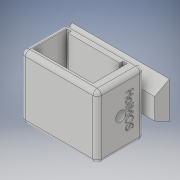
# Autodesk Inventor part: 7.2 Schienenläufer
Saved by Autodesk Inventor 2018.3 (Build 223284000, 284)
## iProperties
Created: 2018-10-11
Part Number: 7.2 Schienenläufer
Material: Generisch
Document SubType Name: Modeling
Designer: pgmadmin
Density: 1 g/cm^3
Appearance: Vorgabe
Author: pgmadmin
Autodesk Inventor part; units mm, degrees
ref_plane "YZ Plane" through (0, 0, 0) normal (1, 0, 0) x (0, 1, 0)
ref_plane "XZ Plane" through (0, 0, 0) normal (0, 1, 0) x (-1, 0, 0)
ref_plane "XY Plane" through (0, 0, 0) normal (0, 0, 1) x (1, 0, 0)
sketch "Skizze1" plane through (0, 0, 0) normal (0, 0, 1) x (1, 0, 0)
  line L0 (-14.1284, 0) -> (-14.1284, 16.2)
  line L1 (-14.1284, 16.2) -> (-12.1284, 16.2)
  line L2 (-12.1284, 16.2) -> (-12.1284, 1.6)
  line L3 (-12.1284, 1.6) -> (12.3716, 1.6)
  line L4 (12.3716, 1.6) -> (12.3716, 16.2)
  line L5 (12.3716, 16.2) -> (14.3716, 16.2)
  line L6 (14.3716, 16.2) -> (14.3716, 0)
  line L7 (14.3716, 0) -> (-14.1284, 0)
  line L8 (-16.6284, 19.2) -> (19.3716, 19.2)
  line L9 (19.3716, 19.2) -> (19.3716, -3)
  line L10 (19.3716, -3) -> (-16.6284, -3)
  line L11 (-16.6284, -3) -> (-16.6284, 19.2)
  line L12 (-12.1284, 14.7) -> (12.3716, 14.7)
  point P0 (0, 0)
  dimension "d1" = 2
  dimension "d3" = 2
  dimension "d4" = 1.6
  dimension "d5" = 3
  dimension "d7" = 2.5
  dimension "d8" = 5
  dimension "d9" = 1.5
  dimension "d26" = 3
  dimension "d27" = 28.5
  dimension "d28" = 16.2
  constraints: 26 end point, 8 perpendicular, 4 point on line, 2 parallel, 1 horizontal, 1 vertical
  measures "d1" distance of L0.end L1.end
  measures "d3" distance of L4.end L5.end
  measures "d4" distance between parallel lines of L3 L7
  measures "d5" distance between parallel lines of L10 L7
  measures "d7" distance between parallel lines of L11 L0
  measures "d8" distance between parallel lines of L9 L6
  measures "d9" distance of L1.end L12.start
  measures "d26" distance between parallel lines of L8 L1
  measures "d27" distance of L6.end L0.start
  measures "d28" distance of L0.start L0.end
extrude "Extrusion1" add sketch "Skizze1" along normal blind 30
fillet "Rundung1" radius 2 12 edges at (19.3716, 19.2, 15) (19.3716, -3, 15) (-16.6284, -3, 15) (-16.6284, 19.2, 15) (1.3716, 19.2, 30) (-16.6284, 8.1, 30) (1.3716, -3, 30) (19.3716, 8.1, 30) (19.3716, 8.1, 0) (1.3716, -3, 0) (1.3716, 19.2, 0) (-16.6284, 8.1, 0)
sketch "Skizze2" plane through (19.3716, -1, 28) normal (1, 0, 0) x (0, 0, -1)
  line L0 (0, 20.2) -> (26, 20.2) projected
  line L1 (8, 20.2) -> (4.25, 27.2)
  line L2 (4.25, 27.2) -> (21.75, 27.2)
  line L3 (21.75, 27.2) -> (18, 20.2)
  line L4 (28, 0) -> (28, 18.2) projected
  point P0 (28, 1)
  dimension "d13" = 10
  dimension "d15" = 7
  dimension "d16" = 3.75
  dimension "d17" = 3.75
  dimension "d18" = 17.5
  dimension "d19" = 10
  constraints: 6 end point, 2 point on line, 1 parallel
  measures "d13" distance of L3.end L1.start
  measures "d15" vertical distance of L1.end L1.start
  measures "d16" horizontal distance of L2.end L3.end
  measures "d17" horizontal distance of L1.start L1.end
  measures "d18" distance of L1.end L2.end
  measures "d19" distance from line of L4 L3.end
extrude "Extrusion2" add sketch "Skizze2" against normal blind 41 and the other way blind 5
sketch "Skizze5" plane through (19.3716, -1, 28) normal (1, 0, 0) x (0, 0, -1)
  circle A0 centre (13, 9.1) radius 2.4
  line L0 (13, 9.1) -> (-2, 9.1)
  line L1 (-2, 18.2) -> (-2, 0) projected
  line L2 (13, 9.1) -> (13, 20.2)
  line L3 (8, 20.2) -> (18, 20.2) projected
  line L4 (13, 9.1) -> (28, 9.1)
  point P0 (28, 1)
  dimension "d31" = 4.8
  dimension "d32" = 90
  dimension "d35" = 15
  constraints: 6 end point, 2 midpoint, 1 centre point, 1 collinear, 1 horizontal, 1 vertical
  measures "d31" diameter of A0
  measures "d32" angle of L2 L0
  measures "d35" distance between parallel lines of L1 L2
extrude "Extrusion5" cut sketch "Skizze5" against normal blind 10
sketch "Skizze6" plane through (19.3716, -1, 28) normal (1, 0, 0) x (0, 0, -1)
  circle A0 centre (13, 9.1) radius 2.4 projected
  line L0 (13, 11.5) -> (-2, 11.5)
  line L1 (-2, 18.2) -> (-2, 0) projected
  line L2 (28, 0) -> (28, 18.2) projected
  line L3 (28, 11.5) -> (13, 11.5)
  line L4 (0, -2) -> (26, -2) projected
  line L5 (6.9088, 11.5) -> (6.4437, 11.5)
  line L6 (6.4437, 11.5) -> (6.4437, 13.2131)
  line L7 (6.4437, 13.2131) -> (4.8327, 13.2131)
  line L8 (4.8327, 13.2131) -> (4.8327, 11.5)
  line L9 (4.8327, 11.5) -> (4.3675, 11.5)
  line L10 (4.3675, 11.5) -> (4.3675, 15)
  line L11 (4.3675, 15) -> (4.8327, 15)
  line L12 (4.8327, 15) -> (4.8327, 13.6272)
  line L13 (4.8327, 13.6272) -> (6.4437, 13.6272)
  line L14 (6.4437, 13.6272) -> (6.4437, 15)
  line L15 (6.4437, 15) -> (6.9088, 15)
  line L16 (6.9088, 15) -> (6.9088, 11.5)
  spline S0 degree 2 poles (9.7423, 12.8132) (9.7423, 12.1495) (9.1041, 11.4263) (8.5709, 11.4263) knots 0 0 0 1 2 2 2
  spline S1 degree 2 poles (8.5709, 11.4263) (8.0235, 11.4263) (7.3967, 12.1722) (7.3967, 12.8132) knots 0 0 0 1 2 2 2
  spline S2 degree 2 poles (7.3967, 12.8132) (7.3967, 13.4712) (8.0434, 14.2002) (8.5709, 14.2002) knots 0 0 0 1 2 2 2
  spline S3 degree 2 poles (8.5709, 14.2002) (9.1041, 14.2002) (9.7423, 13.4741) (9.7423, 12.8132) knots 0 0 0 1 2 2 2
  spline S4 degree 2 poles (9.2857, 12.8132) (9.2857, 13.3237) (8.9141, 13.8201) (8.5709, 13.8201) knots 0 0 0 1 2 2 2
  spline S5 degree 2 poles (8.5709, 13.8201) (8.2277, 13.8201) (7.8533, 13.3237) (7.8533, 12.8132) knots 0 0 0 1 2 2 2
  spline S6 degree 2 poles (7.8533, 12.8132) (7.8533, 12.3169) (8.2277, 11.8063) (8.5709, 11.8063) knots 0 0 0 1 2 2 2
  spline S7 degree 2 poles (8.5709, 11.8063) (8.9113, 11.8063) (9.2857, 12.3083) (9.2857, 12.8132) knots 0 0 0 1 2 2 2
  line L17 (10.6471, 11.5) -> (10.2046, 11.5)
  line L18 (10.2046, 11.5) -> (10.2046, 15.156)
  line L19 (10.2046, 15.156) -> (10.6471, 15.156)
  line L20 (10.6471, 15.156) -> (10.6471, 11.5)
  line L21 (14.3314, 11.5) -> (13.8663, 11.5)
  line L22 (13.8663, 11.5) -> (13.8663, 14.515)
  line L23 (13.8663, 14.515) -> (12.953, 12.4643)
  line L24 (12.953, 12.4643) -> (12.6694, 12.4643)
  line L25 (12.6694, 12.4643) -> (11.7646, 14.515)
  line L26 (11.7646, 14.515) -> (11.7646, 11.5)
  line L27 (11.7646, 11.5) -> (11.3306, 11.5)
  line L28 (11.3306, 11.5) -> (11.3306, 15)
  line L29 (11.3306, 15) -> (11.966, 15)
  line L30 (11.966, 15) -> (12.8395, 13.0515)
  line L31 (12.8395, 13.0515) -> (13.6848, 15)
  line L32 (13.6848, 15) -> (14.3314, 15)
  line L33 (14.3314, 15) -> (14.3314, 11.5)
  spline S8 degree 2 poles (17.5166, 14.6001) (17.7152, 14.3675) (17.9364, 13.6868) (17.9364, 13.25) knots 0 0 0 1 2 2 2
  spline S9 degree 2 poles (17.9364, 13.25) (17.9364, 12.8246) (17.7208, 12.1353) (17.5166, 11.9028) knots 0 0 0 1 2 2 2
  spline S10 degree 2 poles (17.5166, 11.9028) (17.3011, 11.6588) (16.731, 11.4263) (16.3878, 11.4263) knots 0 0 0 1 2 2 2
  spline S11 degree 2 poles (16.3878, 11.4263) (16.0332, 11.4263) (15.466, 11.6673) (15.2589, 11.9028) knots 0 0 0 1 2 2 2
  spline S12 degree 2 poles (15.2589, 11.9028) (15.0575, 12.1353) (14.842, 12.8189) (14.842, 13.25) knots 0 0 0 1 2 2 2
  spline S13 degree 2 poles (14.842, 13.25) (14.842, 13.6896) (15.0604, 14.359) (15.2618, 14.6001) knots 0 0 0 1 2 2 2
  spline S14 degree 2 poles (15.2618, 14.6001) (15.466, 14.8327) (16.0361, 15.0737) (16.3878, 15.0737) knots 0 0 0 1 2 2 2
  spline S15 degree 2 poles (16.3878, 15.0737) (16.7451, 15.0737) (17.3181, 14.8241) (17.5166, 14.6001) knots 0 0 0 1 2 2 2
  spline S16 degree 2 poles (17.4514, 13.25) (17.4514, 13.596) (17.3011, 14.1321) (17.1649, 14.3079) knots 0 0 0 1 2 2 2
  spline S17 degree 2 poles (17.1649, 14.3079) (17.0259, 14.4895) (16.6345, 14.671) (16.3906, 14.671) knots 0 0 0 1 2 2 2
  spline S18 degree 2 poles (16.3906, 14.671) (16.1382, 14.671) (15.7581, 14.4951) (15.6135, 14.3079) knots 0 0 0 1 2 2 2
  spline S19 degree 2 poles (15.6135, 14.3079) (15.4745, 14.1293) (15.327, 13.5904) (15.327, 13.25) knots 0 0 0 1 2 2 2
  spline S20 degree 2 poles (15.327, 13.25) (15.327, 12.5608) (15.9056, 11.829) (16.3906, 11.829) knots 0 0 0 1 2 2 2
  spline S21 degree 2 poles (16.3906, 11.829) (16.8756, 11.829) (17.4514, 12.5608) (17.4514, 13.25) knots 0 0 0 1 2 2 2
  spline S22 degree 2 poles (19.4226, 11.4376) (19.0425, 11.4376) (18.5093, 11.5964) (18.2739, 11.7099) knots 0 0 0 1 2 2 2
  line L34 (18.2739, 11.7099) -> (18.2739, 12.2942)
  line L35 (18.2739, 12.2942) -> (18.3079, 12.2942)
  spline S23 degree 2 poles (18.3079, 12.2942) (18.5377, 12.0786) (19.1191, 11.8404) (19.3886, 11.8404) knots 0 0 0 1 2 2 2
  spline S24 degree 2 poles (19.3886, 11.8404) (19.7743, 11.8404) (20.1686, 12.1609) (20.1686, 12.4246) knots 0 0 0 1 2 2 2
  spline S25 degree 2 poles (20.1686, 12.4246) (20.1686, 12.6345) (19.9615, 12.8955) (19.7374, 12.9607) knots 0 0 0 1 2 2 2
  spline S26 degree 2 poles (19.7374, 12.9607) (19.5758, 13.0061) (19.3063, 13.0685) (19.1049, 13.1195) knots 0 0 0 1 2 2 2
  spline S27 degree 2 poles (19.1049, 13.1195) (18.9234, 13.1677) (18.637, 13.3124) (18.5263, 13.4287) knots 0 0 0 1 2 2 2
  spline S28 degree 2 poles (18.5263, 13.4287) (18.4186, 13.545) (18.2994, 13.857) (18.2994, 14.0612) knots 0 0 0 1 2 2 2
  spline S29 degree 2 poles (18.2994, 14.0612) (18.2994, 14.4866) (18.9631, 15.0624) (19.4765, 15.0624) knots 0 0 0 1 2 2 2
  spline S30 degree 2 poles (19.4765, 15.0624) (19.7715, 15.0624) (20.2934, 14.9461) (20.5174, 14.8355) knots 0 0 0 1 2 2 2
  line L36 (20.5174, 14.8355) -> (20.5174, 14.2796)
  line L37 (20.5174, 14.2796) -> (20.4834, 14.2796)
  spline S31 degree 2 poles (20.4834, 14.2796) (20.316, 14.4327) (19.7942, 14.6596) (19.5077, 14.6596) knots 0 0 0 1 2 2 2
  spline S32 degree 2 poles (19.5077, 14.6596) (19.1844, 14.6596) (18.7844, 14.3562) (18.7844, 14.1094) knots 0 0 0 1 2 2 2
  spline S33 degree 2 poles (18.7844, 14.1094) (18.7844, 13.8882) (19.0199, 13.6244) (19.2411, 13.5648) knots 0 0 0 1 2 2 2
  spline S34 degree 2 poles (19.2411, 13.5648) (19.3886, 13.5251) (19.8169, 13.423) (19.9587, 13.3805) knots 0 0 0 1 2 2 2
  spline S35 degree 2 poles (19.9587, 13.3805) (20.3189, 13.2699) (20.6536, 12.8246) (20.6536, 12.4984) knots 0 0 0 1 2 2 2
  spline S36 degree 2 poles (20.6536, 12.4984) (20.6536, 12.2913) (20.4862, 11.8942) (20.3359, 11.7553) knots 0 0 0 1 2 2 2
  spline S37 degree 2 poles (20.3359, 11.7553) (20.1686, 11.6021) (19.7431, 11.4376) (19.4226, 11.4376) knots 0 0 0 1 2 2 2
  point P0 (28, 1)
  dimension "d36" = 13.5
  constraints: 4 end point, 3 point on line, 2 horizontal, 1 perpendicular, 1 vertical alignment, 1 other
  measures "d36" distance between parallel lines of L4 L0
extrude "Extrusion6" cut sketch "Skizze6" against normal blind 2 contours L0 L6 L7 L8 L10 L11 L12 L13 L14 L15 L16 | S0 S1 L0 | L0 S1 S2 S3 S0 | L0 L18 L19 L20 | S22 L34 L35 S23 S24 S25 S26 S27 S28 S29 S30 L36 L37 S31 S32 S33 S34 S35 S36 S37 L3 | L3 S37 S22 | S11 S12 S13 S14 S15 S8 S9 S10 L3 | L3 S10 S11 | L0 L28 L29 L30 L31 L32 L33 L3 L22 L23 L24 L25 L26
sketch "Skizze7" plane through (-16.6284, -1, 2) normal (-1, 0, 0) x (0, 0, 1)
  line L0 (0, 18.2) -> (0, 0) projected
  line L1 (0, 11.5) -> (25.983, 11.5)
  line L2 (0, -2) -> (26, -2) projected
  line L3 (8.9088, 11.5) -> (8.4437, 11.5)
  line L4 (8.4437, 11.5) -> (8.4437, 13.2131)
  line L5 (8.4437, 13.2131) -> (6.8327, 13.2131)
  line L6 (6.8327, 13.2131) -> (6.8327, 11.5)
  line L7 (6.8327, 11.5) -> (6.3675, 11.5)
  line L8 (6.3675, 11.5) -> (6.3675, 15)
  line L9 (6.3675, 15) -> (6.8327, 15)
  line L10 (6.8327, 15) -> (6.8327, 13.6272)
  line L11 (6.8327, 13.6272) -> (8.4437, 13.6272)
  line L12 (8.4437, 13.6272) -> (8.4437, 15)
  line L13 (8.4437, 15) -> (8.9088, 15)
  line L14 (8.9088, 15) -> (8.9088, 11.5)
  spline S0 degree 2 poles (11.7423, 12.8132) (11.7423, 12.1495) (11.1041, 11.4263) (10.5709, 11.4263) knots 0 0 0 1 2 2 2
  spline S1 degree 2 poles (10.5709, 11.4263) (10.0235, 11.4263) (9.3967, 12.1722) (9.3967, 12.8132) knots 0 0 0 1 2 2 2
  spline S2 degree 2 poles (9.3967, 12.8132) (9.3967, 13.4712) (10.0434, 14.2002) (10.5709, 14.2002) knots 0 0 0 1 2 2 2
  spline S3 degree 2 poles (10.5709, 14.2002) (11.1041, 14.2002) (11.7423, 13.4741) (11.7423, 12.8132) knots 0 0 0 1 2 2 2
  spline S4 degree 2 poles (11.2857, 12.8132) (11.2857, 13.3237) (10.9141, 13.8201) (10.5709, 13.8201) knots 0 0 0 1 2 2 2
  spline S5 degree 2 poles (10.5709, 13.8201) (10.2277, 13.8201) (9.8533, 13.3237) (9.8533, 12.8132) knots 0 0 0 1 2 2 2
  spline S6 degree 2 poles (9.8533, 12.8132) (9.8533, 12.3169) (10.2277, 11.8063) (10.5709, 11.8063) knots 0 0 0 1 2 2 2
  spline S7 degree 2 poles (10.5709, 11.8063) (10.9113, 11.8063) (11.2857, 12.3083) (11.2857, 12.8132) knots 0 0 0 1 2 2 2
  line L15 (12.6471, 11.5) -> (12.2046, 11.5)
  line L16 (12.2046, 11.5) -> (12.2046, 15.156)
  line L17 (12.2046, 15.156) -> (12.6471, 15.156)
  line L18 (12.6471, 15.156) -> (12.6471, 11.5)
  line L19 (16.3314, 11.5) -> (15.8663, 11.5)
  line L20 (15.8663, 11.5) -> (15.8663, 14.515)
  line L21 (15.8663, 14.515) -> (14.953, 12.4643)
  line L22 (14.953, 12.4643) -> (14.6694, 12.4643)
  line L23 (14.6694, 12.4643) -> (13.7646, 14.515)
  line L24 (13.7646, 14.515) -> (13.7646, 11.5)
  line L25 (13.7646, 11.5) -> (13.3306, 11.5)
  line L26 (13.3306, 11.5) -> (13.3306, 15)
  line L27 (13.3306, 15) -> (13.966, 15)
  line L28 (13.966, 15) -> (14.8395, 13.0515)
  line L29 (14.8395, 13.0515) -> (15.6848, 15)
  line L30 (15.6848, 15) -> (16.3314, 15)
  line L31 (16.3314, 15) -> (16.3314, 11.5)
  spline S8 degree 2 poles (19.5166, 14.6001) (19.7152, 14.3675) (19.9364, 13.6868) (19.9364, 13.25) knots 0 0 0 1 2 2 2
  spline S9 degree 2 poles (19.9364, 13.25) (19.9364, 12.8246) (19.7208, 12.1353) (19.5166, 11.9028) knots 0 0 0 1 2 2 2
  spline S10 degree 2 poles (19.5166, 11.9028) (19.3011, 11.6588) (18.731, 11.4263) (18.3878, 11.4263) knots 0 0 0 1 2 2 2
  spline S11 degree 2 poles (18.3878, 11.4263) (18.0332, 11.4263) (17.466, 11.6673) (17.2589, 11.9028) knots 0 0 0 1 2 2 2
  spline S12 degree 2 poles (17.2589, 11.9028) (17.0575, 12.1353) (16.842, 12.8189) (16.842, 13.25) knots 0 0 0 1 2 2 2
  spline S13 degree 2 poles (16.842, 13.25) (16.842, 13.6896) (17.0604, 14.359) (17.2618, 14.6001) knots 0 0 0 1 2 2 2
  spline S14 degree 2 poles (17.2618, 14.6001) (17.466, 14.8327) (18.0361, 15.0737) (18.3878, 15.0737) knots 0 0 0 1 2 2 2
  spline S15 degree 2 poles (18.3878, 15.0737) (18.7451, 15.0737) (19.3181, 14.8241) (19.5166, 14.6001) knots 0 0 0 1 2 2 2
  spline S16 degree 2 poles (19.4514, 13.25) (19.4514, 13.596) (19.3011, 14.1321) (19.1649, 14.3079) knots 0 0 0 1 2 2 2
  spline S17 degree 2 poles (19.1649, 14.3079) (19.0259, 14.4895) (18.6345, 14.671) (18.3906, 14.671) knots 0 0 0 1 2 2 2
  spline S18 degree 2 poles (18.3906, 14.671) (18.1382, 14.671) (17.7581, 14.4951) (17.6135, 14.3079) knots 0 0 0 1 2 2 2
  spline S19 degree 2 poles (17.6135, 14.3079) (17.4745, 14.1293) (17.327, 13.5904) (17.327, 13.25) knots 0 0 0 1 2 2 2
  spline S20 degree 2 poles (17.327, 13.25) (17.327, 12.5608) (17.9056, 11.829) (18.3906, 11.829) knots 0 0 0 1 2 2 2
  spline S21 degree 2 poles (18.3906, 11.829) (18.8756, 11.829) (19.4514, 12.5608) (19.4514, 13.25) knots 0 0 0 1 2 2 2
  spline S22 degree 2 poles (21.4226, 11.4376) (21.0425, 11.4376) (20.5093, 11.5964) (20.2739, 11.7099) knots 0 0 0 1 2 2 2
  line L32 (20.2739, 11.7099) -> (20.2739, 12.2942)
  line L33 (20.2739, 12.2942) -> (20.3079, 12.2942)
  spline S23 degree 2 poles (20.3079, 12.2942) (20.5377, 12.0786) (21.1191, 11.8404) (21.3886, 11.8404) knots 0 0 0 1 2 2 2
  spline S24 degree 2 poles (21.3886, 11.8404) (21.7743, 11.8404) (22.1686, 12.1609) (22.1686, 12.4246) knots 0 0 0 1 2 2 2
  spline S25 degree 2 poles (22.1686, 12.4246) (22.1686, 12.6345) (21.9615, 12.8955) (21.7374, 12.9607) knots 0 0 0 1 2 2 2
  spline S26 degree 2 poles (21.7374, 12.9607) (21.5758, 13.0061) (21.3063, 13.0685) (21.1049, 13.1195) knots 0 0 0 1 2 2 2
  spline S27 degree 2 poles (21.1049, 13.1195) (20.9234, 13.1677) (20.637, 13.3124) (20.5263, 13.4287) knots 0 0 0 1 2 2 2
  spline S28 degree 2 poles (20.5263, 13.4287) (20.4186, 13.545) (20.2994, 13.857) (20.2994, 14.0612) knots 0 0 0 1 2 2 2
  spline S29 degree 2 poles (20.2994, 14.0612) (20.2994, 14.4866) (20.9631, 15.0624) (21.4765, 15.0624) knots 0 0 0 1 2 2 2
  spline S30 degree 2 poles (21.4765, 15.0624) (21.7715, 15.0624) (22.2934, 14.9461) (22.5174, 14.8355) knots 0 0 0 1 2 2 2
  line L34 (22.5174, 14.8355) -> (22.5174, 14.2796)
  line L35 (22.5174, 14.2796) -> (22.4834, 14.2796)
  spline S31 degree 2 poles (22.4834, 14.2796) (22.316, 14.4327) (21.7942, 14.6596) (21.5077, 14.6596) knots 0 0 0 1 2 2 2
  spline S32 degree 2 poles (21.5077, 14.6596) (21.1844, 14.6596) (20.7844, 14.3562) (20.7844, 14.1094) knots 0 0 0 1 2 2 2
  spline S33 degree 2 poles (20.7844, 14.1094) (20.7844, 13.8882) (21.0199, 13.6244) (21.2411, 13.5648) knots 0 0 0 1 2 2 2
  spline S34 degree 2 poles (21.2411, 13.5648) (21.3886, 13.5251) (21.8169, 13.423) (21.9587, 13.3805) knots 0 0 0 1 2 2 2
  spline S35 degree 2 poles (21.9587, 13.3805) (22.3189, 13.2699) (22.6536, 12.8246) (22.6536, 12.4984) knots 0 0 0 1 2 2 2
  spline S36 degree 2 poles (22.6536, 12.4984) (22.6536, 12.2913) (22.4862, 11.8942) (22.3359, 11.7553) knots 0 0 0 1 2 2 2
  spline S37 degree 2 poles (22.3359, 11.7553) (22.1686, 11.6021) (21.7431, 11.4376) (21.4226, 11.4376) knots 0 0 0 1 2 2 2
  point P0 (-2, 1)
  dimension "d39" = 13.5
  constraints: 2 end point, 2 horizontal, 1 point on line
  measures "d39" distance between parallel lines of L2 L1
extrude "Extrusion7" cut sketch "Skizze7" against normal blind 2 contours L8 L9 L10 L11 L12 L13 L14 L1 L4 L5 L6 | S22 L32 L33 S23 S24 S25 S26 S27 S28 S29 S30 L34 L35 S31 S32 S33 S34 S35 S36 S37 L1 | L1 S37 S22 | S11 S12 S13 S14 S15 S8 S9 S10 L1 | L1 S10 S11 | L26 L27 L28 L29 L30 L31 L1 L20 L21 L22 L23 L24 | L16 L17 L18 L1 | S1 S2 S3 S0 L1 | L1 S0 S1
